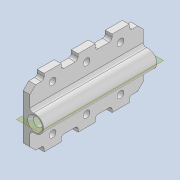
# Autodesk Inventor part: bl_tube_hn_1
Saved by Autodesk Inventor 2020 (Build 240168000, 168)
## iProperties
Created: 2021-10-07
Part Number: bl_tube_hn_1
Material: Generic
Document SubType Name: Modeling
Designer: Shuang Peng
Density: 1 g/cm^3
Appearance: Default
Author: Shuang Peng
Autodesk Inventor part; units mm, degrees
ref_plane "YZ Plane" through (0, 0, 0) normal (1, 0, 0) x (0, 1, 0)
ref_plane "XZ Plane" through (0, 0, 0) normal (0, 1, 0) x (-1, 0, 0)
ref_plane "XY Plane" through (0, 0, 0) normal (0, 0, 1) x (1, 0, 0)
sketch "Sketch1" plane through (0, 0, 0) normal (0, 0, 1) x (1, 0, 0)
  circle A0 centre (0, 0) radius 0.8 projected
  circle A1 centre (0, 0) radius 0.4 projected
  circle A2 centre (0, 0) radius 0.8
  circle A3 centre (0, 0) radius 1.5
  line L0 (0, 0) -> (-1.5, 0)
  line L1 (-0.8, 0) -> (-1.5, 0)
  line L2 (-2.1, 5) -> (-0.9, 5)
  line L3 (-0.9, 5) -> (-0.9, -5)
  line L4 (-0.9, -5) -> (-2.1, -5)
  line L5 (-2.1, -5) -> (-2.1, 5)
  line L6 (-2.1, 5) -> (-0.9, -5) construction
  line L7 (-0.9, 5) -> (-2.1, -5) construction
  point P0 (-0.9, -1.2)
  point P1 (-0.9, 1.2)
  dimension "d0" = 1.6
  dimension "d1" = 3
  dimension "d2" = 1.2
  dimension "d3" = 10
  constraints: 16 end point, 3 parallel, 2 coincident, 2 midpoint, 1 collinear, 1 horizontal, 1 horizontal alignment, 1 perpendicular, 1 point on line, 5 other
  measures "d2" distance of L2.start L2.end
  measures "d3" distance of L2.end L3.end
extrude "Extrusion1" add sketch "Sketch1" against normal blind 20 contours A3 L3 | L3 L0 A3 | A3 L3 L4 L5 L2 | A3 L0 L3
fillet "Fillet1" radius 0.5 2 edges at (-0.9, -1.2, -10) (-0.9, 1.2, -10)
chamfer "Chamfer1" distance 0.5 angle 45 2 edges at (-0.8, 0, -20) (-0.8, 0, 0)
sketch "Sketch2" plane through (-0.9, 5, 0) normal (1, 0, 0) x (0, 0, -1)
  line L0 (20, -3.0404) -> (0, -3.0404) projected
  line L1 (20, 0) -> (20, -3.0404) projected
  line L2 (0, 0) -> (20, 0) projected
  line L3 (0, -3.0404) -> (0, 0) projected
  line L4 (20, 0) -> (20, -3.0404) projected
  line L5 (20, 0) -> (20, -1)
  line L6 (20, -1) -> (16, -1)
  line L7 (16, -1) -> (10, -1)
  line L8 (10, -1) -> (4, -1)
  line L9 (4, -1) -> (0, -1)
  line L10 (0, -3.0404) -> (0, 0) projected
  circle A0 centre (16, -1) radius 0.6
  circle A1 centre (10, -1) radius 0.6
  circle A2 centre (4, -1) radius 0.6
  point P0 (0, -5)
  dimension "d10" = 1
  dimension "d11" = 4
  dimension "d12" = 6
  dimension "d13" = 6
  dimension "d14" = 1.2
  dimension "d15" = 1.2
  dimension "d16" = 1.2
  constraints: 10 end point, 4 point on line, 3 centre point, 3 coincident, 2 perpendicular
  measures "d10" distance of L1.start L5.end
  measures "d11" distance of L5.end L6.end
  measures "d12" distance of L6.end L7.end
  measures "d13" distance of L7.end L8.end
  measures "d14" diameter of A0
  measures "d15" diameter of A1
  measures "d16" diameter of A2
extrude "Extrusion2" cut sketch "Sketch2" against normal blind 20 contours A0 L7 L6 | L6 L7 A0 | A2 L8 L9 | L9 L8 A2 | A1 L8 L7 | L7 L8 A1
sketch "Sketch3" plane through (-0.9, 5, 0) normal (1, 0, 0) x (0, 0, -1)
  circle A0 centre (4, -1) radius 0.6 projected
  circle A1 centre (10, -1) radius 0.6 projected
  circle A2 centre (16, -1) radius 0.6 projected
  line L0 (20, -3.0404) -> (0, -3.0404) projected
  line L1 (20, 0) -> (20, -3.0404) projected
  line L2 (0, 0) -> (20, 0) projected
  line L3 (0, -3.0404) -> (0, 0) projected
  line L4 (17.5, -3) -> (17.5, 1)
  line L5 (17.5, 1) -> (14.5, 1)
  line L6 (14.5, 1) -> (14.5, -3)
  line L7 (14.5, -3) -> (17.5, -3)
  line L8 (17.5, -3) -> (14.5, 1) construction
  line L9 (17.5, 1) -> (14.5, -3) construction
  line L10 (11.5, 1) -> (11.5, -3)
  line L11 (11.5, -3) -> (8.5, -3)
  line L12 (8.5, -3) -> (8.5, 1)
  line L13 (8.5, 1) -> (11.5, 1)
  line L14 (11.5, 1) -> (8.5, -3) construction
  line L15 (11.5, -3) -> (8.5, 1) construction
  line L16 (5.5, 1) -> (5.5, -3)
  line L17 (5.5, -3) -> (2.5, -3)
  line L18 (2.5, -3) -> (2.5, 1)
  line L19 (2.5, 1) -> (5.5, 1)
  line L20 (5.5, 1) -> (2.5, -3) construction
  line L21 (5.5, -3) -> (2.5, 1) construction
  point P0 (0, -5)
  point P1 (2.5, 0)
  point P2 (5.5, 0)
  point P3 (8.5, 0)
  point P4 (11.5, 0)
  point P5 (14.5, 0)
  point P6 (17.5, 0)
  dimension "d19" = 4
  dimension "d20" = 3
  dimension "d21" = 4
  dimension "d22" = 3
  dimension "d23" = 4
  dimension "d24" = 3
  constraints: 36 end point, 6 midpoint, 6 parallel, 4 perpendicular, 2 vertical
  measures "d19" distance of L4.start L4.end
  measures "d20" distance of L5.end L4.end
  measures "d21" distance of L10.start L10.end
  measures "d22" distance of L10.end L11.end
  measures "d23" distance of L16.start L16.end
  measures "d24" distance of L16.end L17.end
extrude "Extrusion3" add sketch "Sketch3" against normal up to surface (1.2 mm away) contours L2 L6 L5 L4 | L18 L19 L16 L2 | L2 L12 L13 L10
ref_plane "Work Plane1" through (-2.1, 0, 0) normal (0, -1, 0) x (1, 0, 0)
mirror "Mirror1" about plane through (-2.1, 0, 0) normal (0, -1, 0) of "Extrusion2", "Extrusion3"
fillet "Fillet2" radius 0.5 12 edges at (-1.5, 5, -17.5) (-1.5, 5, -14.5) (-1.5, 5, -11.5) (-1.5, 5, -8.5) (-1.5, 5, -5.5) (-1.5, 5, -2.5) (-1.5, -5, -2.5) (-1.5, -5, -5.5) (-1.5, -5, -8.5) (-1.5, -5, -11.5) (-1.5, -5, -14.5) (-1.5, -5, -17.5)
chamfer "Chamfer2" distance 1 angle 45 4 edges at (-1.5, 5, -20) (-1.5, -5, -20) (-1.5, 5, 0) (-1.5, -5, 0)
body "Solid1"
